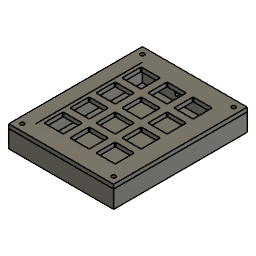
Macropad (Autodesk Fusion 360 design; units mm, degrees)
Autodesk Fusion 360 part; units mm, degrees
sketch "Sketch1" plane through (0, 0, 0) normal (0, 1, 0) x (1, 0, 0)
  line L0 (0, 0) -> (56.985, 0)
  line L1 (56.985, 0) -> (56.985, 78.065)
  line L2 (56.985, 78.065) -> (0, 78.065)
  line L3 (0, 78.065) -> (0, 0)
  line L4 (66.985, -10) -> (66.985, 88.065)
  line L5 (66.985, 88.065) -> (-10, 88.065)
  line L6 (-10, 88.065) -> (-10, -10)
  line L7 (-10, -10) -> (66.985, -10)
  circle A0 centre (-5, 83.065) radius 1.45
  circle A1 centre (-5, -5) radius 1.45
  circle A2 centre (61.985, -5) radius 1.45
  circle A3 centre (61.985, 83.065) radius 1.45
  dimension "d4" = 56.985
  dimension "d5" = 78.065
  dimension "d6" = 10
  dimension "d9" = 2.9
  dimension "d12" = 2.9
  dimension "d15" = 2.9
  dimension "d18" = 2.9
  constraint horizontal L0
  constraint vertical L1
  constraint horizontal L2
  constraint vertical L3
  constraint coincident L0.start L3.end
  measures "d4" distance of L0.start L0.end
  measures "d5" distance of L0.start L2.end
  measures "d9" diameter of A0
  measures "d12" diameter of A1
  measures "d15" diameter of A2
  measures "d18" diameter of A3
extrude "Extrude1" add sketch "Sketch1" along normal blind 3 contours L0 L1 L2 L3 | L4 L5 L6 L7 picked at (18.995, 52.043333) picked at (60.825164, 26.021667) makes body 1
extrude "Extrude2" cut sketch "Sketch1" along normal blind 13 bodies 1
extrude "Extrude3" add sketch "Sketch1" along normal blind 13 bodies 1
move_body "Align1" bodies 1 to x (1, 0, 0) y (0, 1, 0) z (0, 0, 1) at (0, 0, 0)
move_body "Align2" bodies 1 to x (1, 0, 0) y (0, 1, 0) z (0, 0, 1) at (0, 0, 0)
move_body "Align3" bodies 1 to x (1, 0, 0) y (0, 1, 0) z (0, 0, 1) at (-28.4925, -5.248423, 39.0325)
sketch "plate-2026-03-13T21_26_14.409Z" plane through (0, 7.751577, 0) normal (0, 1, 0) x (1, 0, 0)
  line L0 (-25.209257, 35.572548) -> (-12.209257, 35.572548)
  line L1 (-25.209257, 21.572548) -> (-12.209257, 21.572548)
  line L2 (-25.709257, 35.072548) -> (-25.709257, 22.072548)
  line L3 (-11.709257, 35.072548) -> (-11.709257, 22.072548)
  arc A0 (-25.209257, 35.572548) -> (-25.709257, 35.072548) centre (-25.209257, 35.072548) ccw
  arc A1 (-11.709257, 35.072548) -> (-12.209257, 35.572548) centre (-12.209257, 35.072548) ccw
  arc A2 (-25.709257, 22.072548) -> (-25.209257, 21.572548) centre (-25.209257, 22.072548) ccw
  arc A3 (-12.209257, 21.572548) -> (-11.709257, 22.072548) centre (-12.209257, 22.072548) ccw
  line L4 (-6.159257, 35.572548) -> (6.840743, 35.572548)
  line L5 (-6.159257, 21.572548) -> (6.840743, 21.572548)
  line L6 (-6.659257, 35.072548) -> (-6.659257, 22.072548)
  line L7 (7.340743, 35.072548) -> (7.340743, 22.072548)
  arc A4 (-6.159257, 35.572548) -> (-6.659257, 35.072548) centre (-6.159257, 35.072548) ccw
  arc A5 (7.340743, 35.072548) -> (6.840743, 35.572548) centre (6.840743, 35.072548) ccw
  arc A6 (-6.659257, 22.072548) -> (-6.159257, 21.572548) centre (-6.159257, 22.072548) ccw
  arc A7 (6.840743, 21.572548) -> (7.340743, 22.072548) centre (6.840743, 22.072548) ccw
  line L8 (12.890743, 35.572548) -> (25.890743, 35.572548)
  line L9 (12.890743, 21.572548) -> (25.890743, 21.572548)
  line L10 (12.390743, 35.072548) -> (12.390743, 22.072548)
  line L11 (26.390743, 35.072548) -> (26.390743, 22.072548)
  arc A8 (12.890743, 35.572548) -> (12.390743, 35.072548) centre (12.890743, 35.072548) ccw
  arc A9 (26.390743, 35.072548) -> (25.890743, 35.572548) centre (25.890743, 35.072548) ccw
  arc A10 (12.390743, 22.072548) -> (12.890743, 21.572548) centre (12.890743, 22.072548) ccw
  arc A11 (25.890743, 21.572548) -> (26.390743, 22.072548) centre (25.890743, 22.072548) ccw
  line L12 (-25.209257, 16.522548) -> (-12.209257, 16.522548)
  line L13 (-25.209257, 2.522548) -> (-12.209257, 2.522548)
  line L14 (-25.709257, 16.022548) -> (-25.709257, 3.022548)
  line L15 (-11.709257, 16.022548) -> (-11.709257, 3.022548)
  arc A12 (-25.209257, 16.522548) -> (-25.709257, 16.022548) centre (-25.209257, 16.022548) ccw
  arc A13 (-11.709257, 16.022548) -> (-12.209257, 16.522548) centre (-12.209257, 16.022548) ccw
  arc A14 (-25.709257, 3.022548) -> (-25.209257, 2.522548) centre (-25.209257, 3.022548) ccw
  arc A15 (-12.209257, 2.522548) -> (-11.709257, 3.022548) centre (-12.209257, 3.022548) ccw
  line L16 (-6.159257, 16.522548) -> (6.840743, 16.522548)
  line L17 (-6.159257, 2.522548) -> (6.840743, 2.522548)
  line L18 (-6.659257, 16.022548) -> (-6.659257, 3.022548)
  line L19 (7.340743, 16.022548) -> (7.340743, 3.022548)
  arc A16 (-6.159257, 16.522548) -> (-6.659257, 16.022548) centre (-6.159257, 16.022548) ccw
  arc A17 (7.340743, 16.022548) -> (6.840743, 16.522548) centre (6.840743, 16.022548) ccw
  arc A18 (-6.659257, 3.022548) -> (-6.159257, 2.522548) centre (-6.159257, 3.022548) ccw
  arc A19 (6.840743, 2.522548) -> (7.340743, 3.022548) centre (6.840743, 3.022548) ccw
  line L20 (12.890743, 16.522548) -> (25.890743, 16.522548)
  line L21 (12.890743, 2.522548) -> (25.890743, 2.522548)
  line L22 (12.390743, 16.022548) -> (12.390743, 3.022548)
  line L23 (26.390743, 16.022548) -> (26.390743, 3.022548)
  arc A20 (12.890743, 16.522548) -> (12.390743, 16.022548) centre (12.890743, 16.022548) ccw
  arc A21 (26.390743, 16.022548) -> (25.890743, 16.522548) centre (25.890743, 16.022548) ccw
  arc A22 (12.390743, 3.022548) -> (12.890743, 2.522548) centre (12.890743, 3.022548) ccw
  arc A23 (25.890743, 2.522548) -> (26.390743, 3.022548) centre (25.890743, 3.022548) ccw
  line L24 (-25.209257, -2.527452) -> (-12.209257, -2.527452)
  line L25 (-25.209257, -16.527452) -> (-12.209257, -16.527452)
  line L26 (-25.709257, -3.027452) -> (-25.709257, -16.027452)
  line L27 (-11.709257, -3.027452) -> (-11.709257, -16.027452)
  arc A24 (-25.209257, -2.527452) -> (-25.709257, -3.027452) centre (-25.209257, -3.027452) ccw
  arc A25 (-11.709257, -3.027452) -> (-12.209257, -2.527452) centre (-12.209257, -3.027452) ccw
  arc A26 (-25.709257, -16.027452) -> (-25.209257, -16.527452) centre (-25.209257, -16.027452) ccw
  arc A27 (-12.209257, -16.527452) -> (-11.709257, -16.027452) centre (-12.209257, -16.027452) ccw
  line L28 (-6.159257, -2.527452) -> (6.840743, -2.527452)
  line L29 (-6.159257, -16.527452) -> (6.840743, -16.527452)
  line L30 (-6.659257, -3.027452) -> (-6.659257, -16.027452)
  line L31 (7.340743, -3.027452) -> (7.340743, -16.027452)
  arc A28 (-6.159257, -2.527452) -> (-6.659257, -3.027452) centre (-6.159257, -3.027452) ccw
  arc A29 (7.340743, -3.027452) -> (6.840743, -2.527452) centre (6.840743, -3.027452) ccw
  arc A30 (-6.659257, -16.027452) -> (-6.159257, -16.527452) centre (-6.159257, -16.027452) ccw
  arc A31 (6.840743, -16.527452) -> (7.340743, -16.027452) centre (6.840743, -16.027452) ccw
  line L32 (12.890743, -2.527452) -> (25.890743, -2.527452)
  line L33 (12.890743, -16.527452) -> (25.890743, -16.527452)
  line L34 (12.390743, -3.027452) -> (12.390743, -16.027452)
  line L35 (26.390743, -3.027452) -> (26.390743, -16.027452)
  arc A32 (12.890743, -2.527452) -> (12.390743, -3.027452) centre (12.890743, -3.027452) ccw
  arc A33 (26.390743, -3.027452) -> (25.890743, -2.527452) centre (25.890743, -3.027452) ccw
  arc A34 (12.390743, -16.027452) -> (12.890743, -16.527452) centre (12.890743, -16.027452) ccw
  arc A35 (25.890743, -16.527452) -> (26.390743, -16.027452) centre (25.890743, -16.027452) ccw
  line L36 (12.890743, -2.527452) -> (25.890743, -2.527452)
  line L37 (12.890743, -16.527452) -> (25.890743, -16.527452)
  line L38 (12.390743, -3.027452) -> (12.390743, -16.027452)
  line L39 (26.390743, -3.027452) -> (26.390743, -16.027452)
  arc A36 (12.890743, -2.527452) -> (12.390743, -3.027452) centre (12.890743, -3.027452) ccw
  arc A37 (26.390743, -3.027452) -> (25.890743, -2.527452) centre (25.890743, -3.027452) ccw
  arc A38 (12.390743, -16.027452) -> (12.890743, -16.527452) centre (12.890743, -16.027452) ccw
  arc A39 (25.890743, -16.527452) -> (26.390743, -16.027452) centre (25.890743, -16.027452) ccw
  line L40 (-25.209257, -21.577452) -> (-12.209257, -21.577452)
  line L41 (-25.209257, -35.577452) -> (-12.209257, -35.577452)
  line L42 (-25.709257, -22.077452) -> (-25.709257, -35.077452)
  line L43 (-11.709257, -22.077452) -> (-11.709257, -35.077452)
  arc A40 (-25.209257, -21.577452) -> (-25.709257, -22.077452) centre (-25.209257, -22.077452) ccw
  arc A41 (-11.709257, -22.077452) -> (-12.209257, -21.577452) centre (-12.209257, -22.077452) ccw
  arc A42 (-25.709257, -35.077452) -> (-25.209257, -35.577452) centre (-25.209257, -35.077452) ccw
  arc A43 (-12.209257, -35.577452) -> (-11.709257, -35.077452) centre (-12.209257, -35.077452) ccw
  line L44 (-6.159257, -21.577452) -> (6.840743, -21.577452)
  line L45 (-6.159257, -35.577452) -> (6.840743, -35.577452)
  line L46 (-6.659257, -22.077452) -> (-6.659257, -35.077452)
  line L47 (7.340743, -22.077452) -> (7.340743, -35.077452)
  arc A44 (-6.159257, -21.577452) -> (-6.659257, -22.077452) centre (-6.159257, -22.077452) ccw
  arc A45 (7.340743, -22.077452) -> (6.840743, -21.577452) centre (6.840743, -22.077452) ccw
  arc A46 (-6.659257, -35.077452) -> (-6.159257, -35.577452) centre (-6.159257, -35.077452) ccw
  arc A47 (6.840743, -35.577452) -> (7.340743, -35.077452) centre (6.840743, -35.077452) ccw
  line L48 (12.890743, -21.577452) -> (25.890743, -21.577452)
  line L49 (12.890743, -35.577452) -> (25.890743, -35.577452)
  line L50 (12.390743, -22.077452) -> (12.390743, -35.077452)
  line L51 (26.390743, -22.077452) -> (26.390743, -35.077452)
  arc A48 (12.890743, -21.577452) -> (12.390743, -22.077452) centre (12.890743, -22.077452) ccw
  arc A49 (26.390743, -22.077452) -> (25.890743, -21.577452) centre (25.890743, -22.077452) ccw
  arc A50 (12.390743, -35.077452) -> (12.890743, -35.577452) centre (12.890743, -35.077452) ccw
  arc A51 (25.890743, -35.577452) -> (26.390743, -35.077452) centre (25.890743, -35.077452) ccw
  line L52 (-28.234257, -39.156471) -> (28.915743, -39.156471)
  line L53 (-28.234257, 39.046164) -> (28.915743, 39.046164)
  line L54 (-28.234257, -39.156471) -> (-28.234257, 39.046164)
  line L55 (28.915743, -39.156471) -> (28.915743, 39.046164)
move_body "Move1" bodies 1 to x (1, 0, 0) y (0, 1, 0) z (0, 0, 1) at (0.258, 0, 0)
extrude "Extrude4" add sketch "plate-2026-03-13T21_26_14.409Z" 1 faces at (32.590664, 7.751577, 13.010833) along normal blind 3 separate body on bodies 1 makes body 2
sketch "Sketch3" plane through (0, 0, -49.0325) normal (0, 0, -1) x (-1, 0, 0)
  line L0 (-38.7505, -5.248423) -> (38.2345, -5.248423)
  line L1 (38.2345, -5.248423) -> (38.2345, 7.751577)
  line L2 (38.2345, 7.751577) -> (-38.7505, 7.751577)
  line L3 (-38.7505, 7.751577) -> (-38.7505, -5.248423)
  line L4 (-3.758, 1.551577) -> (3.242, 1.551577)
  line L5 (4.242, 2.551577) -> (4.242, 3.551577)
  line L6 (3.242, 4.551577) -> (-3.758, 4.551577)
  line L7 (-4.758, 3.551577) -> (-4.758, 2.551577)
  arc A0 (4.242, 3.551577) -> (3.242, 4.551577) centre (3.242, 3.551577) ccw
  arc A1 (3.242, 1.551577) -> (4.242, 2.551577) centre (3.242, 2.551577) ccw
  arc A2 (-3.758, 4.551577) -> (-4.758, 3.551577) centre (-3.758, 3.551577) ccw
  arc A3 (-4.758, 2.551577) -> (-3.758, 1.551577) centre (-3.758, 2.551577) ccw
  dimension "d34" = 1
  dimension "d35" = 1
  dimension "d36" = 1
  dimension "d37" = 1
  constraint horizontal L4
  constraint vertical L5
  constraint horizontal L6
  constraint vertical L7
  constraint tangent L6 A0
  constraint tangent L5 A0
  constraint tangent L4 A1
  constraint tangent L5 A1
  constraint tangent L7 A2
  constraint tangent L6 A2
  constraint tangent L7 A3
  constraint tangent L4 A3
  measures "d34" radius of A0
  measures "d35" radius of A1
  measures "d36" radius of A2
  measures "d37" radius of A3
extrude "Extrude5" cut sketch "Sketch3" against normal blind 17 contours L4 L5 L6 L7 A0 A1 A2 A3 picked at (0.908667, 2.551577) bodies 1
sketch "Sketch4" plane through (0, 0, -49.0325) normal (0, 0, -1) x (-1, 0, 0)
  line L0 (3.242, 1.551577) -> (-3.758, 1.551577)
  arc A0 (-4.758, 2.551577) -> (-3.758, 1.551577) centre (-3.758, 2.551577) ccw
  line L1 (-4.758, 2.551577) -> (-4.758, 3.551577)
  arc A1 (-3.758, 4.551577) -> (-4.758, 3.551577) centre (-3.758, 3.551577) ccw
  line L2 (-3.758, 4.551577) -> (3.242, 4.551577)
  arc A2 (4.242, 3.551577) -> (3.242, 4.551577) centre (3.242, 3.551577) ccw
  line L3 (4.242, 3.551577) -> (4.242, 2.551577)
  arc A3 (3.242, 1.551577) -> (4.242, 2.551577) centre (3.242, 2.551577) ccw
  line L4 (-38.7505, -5.248423) -> (38.2345, -5.248423)
  line L5 (38.2345, -5.248423) -> (38.2345, 7.751577)
  line L6 (38.2345, 7.751577) -> (-38.7505, 7.751577)
  line L7 (-38.7505, 7.751577) -> (-38.7505, -5.248423)
  arc A4 (7.242, 3.551577) -> (3.242, 7.551577) centre (3.242, 3.551577) ccw
  line L8 (-3.758, 7.551577) -> (3.242, 7.551577)
  arc A5 (-3.758, 7.551577) -> (-7.758, 3.551577) centre (-3.758, 3.551577) ccw
  line L9 (-7.758, 2.551577) -> (-7.758, 3.551577)
  arc A6 (-7.758, 2.551577) -> (-3.758, -1.448423) centre (-3.758, 2.551577) ccw
  line L10 (3.242, -1.448423) -> (-3.758, -1.448423)
  arc A7 (3.242, -1.448423) -> (7.242, 2.551577) centre (3.242, 2.551577) ccw
  line L11 (7.242, 3.551577) -> (7.242, 2.551577)
  dimension "d40" = -3
extrude "Extrude6" cut sketch "Sketch4" against normal blind 7 contours A4 L8 A5 L9 A6 L10 A7 L11 picked at (-1.424667, -0.448423) bodies 1
